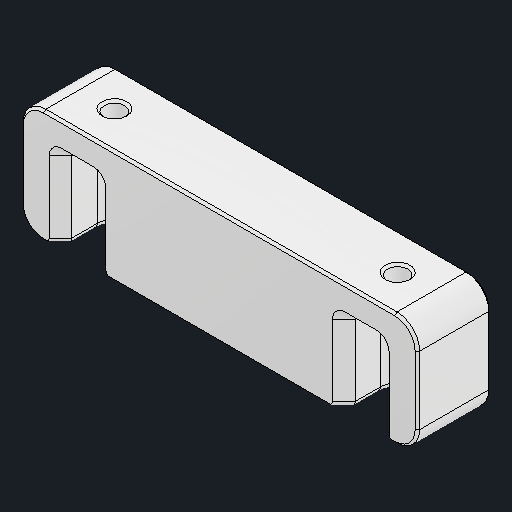
# Autodesk Inventor part: panel-mout
Saved by Autodesk Inventor 2026 (Build 300175050, 175E)
## iProperties
Created: 2026-03-04
Part Number: panel-mout
Material: ABS Plastic
Document SubType Name: Modeling
Designer: kuzmin
Density: 1.06 g/cm^3
Appearance: Smooth - White
Author: kuzmin
Autodesk Inventor part; units mm, degrees
ref_plane "YZ Plane" through (0, 0, 0) normal (1, 0, 0) x (0, 1, 0)
ref_plane "XZ Plane" through (0, 0, 0) normal (0, 1, 0) x (-1, 0, 0)
ref_plane "XY Plane" through (0, 0, 0) normal (0, 0, 1) x (1, 0, 0)
sketch "Sketch1" plane through (0, 0, 0) normal (0, 0, 1) x (1, 0, 0)
  line L0 (-35, 10) -> (35, 10)
  line L1 (35, 10) -> (35, -10)
  line L2 (35, -10) -> (-35, -10)
  line L3 (-35, -10) -> (-35, 10)
  point P0 (0, 0)
  point P1 (0, 10)
  point P2 (35, 0)
  dimension "d0" = 70
  dimension "d1" = 20
  constraints: 8 end point, 2 midpoint, 2 parallel, 1 horizontal, 1 horizontal alignment, 1 perpendicular, 1 vertical alignment
  measures "d0" distance of L0.start L0.end
  measures "d1" distance of L0.end L1.end
extrude "Extrusion1" add sketch "Sketch1" along normal mid plane 13
sketch "Sketch2" plane through (-35, 10, -6.5) normal (0, 1, 0) x (1, 0, 0)
  line L0 (10, -6.5) -> (60, -6.5) construction
  line L1 (0, 0) -> (70, 0) projected
  point P0 (35, -6.5)
  point P1 (35, 0)
  dimension "d4" = 50
  constraints: 2 coincident, 2 end point, 1 horizontal, 1 midpoint, 2 other
  measures "d4" distance of L0.start L0.end
hole "Hole1" at (-25, 10, 0) at (25, 10, 0) direction (0, -1, 0) diameter 3.6 end through all counterbore diameter 6 counterbore depth 13.8
sketch "Sketch3" plane through (-35, 10, 6.5) normal (0, 1, 0) x (1, 0, 0)
  circle A0 centre (10, 6.5) radius 3 projected
  circle A1 centre (60, 6.5) radius 3 projected
  line L0 (7, 6.5) -> (7, 13)
  line L1 (0, 13) -> (70, 13) projected
  line L2 (13, 6.5) -> (13, 13)
  line L3 (57, 6.5) -> (57, 13)
  line L4 (63, 6.5) -> (63, 13)
  point P0 (35, 6.5)
  constraints: 8 end point, 4 point on circle, 4 point on line, 3 parallel, 1 vertical
extrude "Extrusion2" cut sketch "Sketch3" against normal up to surface (13.8 mm away) contours A0 L0 L1 L2 | A1 L3 L1 L4
fillet "Fillet1" radius 0.2 6 edges at (-25, -3.8, 3) (-22, -3.8, -3.25) (-28, -3.8, -3.25) (25, -3.8, 3) (28, -3.8, -3.25) (22, -3.8, -3.25)
chamfer "Chamfer1" distance 2 angle 45 10 edges at (-28, 3.2, -6.5) (-27.9414, -3.7414, -6.5) (-25, -3.8, -6.5) (-22.0586, -3.7414, -6.5) (-22, 3.2, -6.5) (25, -3.8, -6.5) (27.9414, -3.7414, -6.5) (28, 3.2, -6.5) (22.0586, -3.7414, -6.5) (22, 3.2, -6.5)
fillet "Fillet2" radius 4 4 edges at (-35, 10, 0) (35, 10, 0) (35, -10, 0) (-35, -10, 0)
chamfer "Chamfer2" distance 0.4 angle 45 4 edges at (-25, -10, -1.8) (25, -10, -1.8) (25, -3.8, -1.8) (-25, -3.8, -1.8)
chamfer "Chamfer3" distance 0.4 angle 45 18 edges at (0, -10, -6.5) (-33.8284, -8.8284, -6.5) (-35, 0, -6.5) (-33.8284, 8.8284, -6.5) (-30.5, 10, -6.5) (33.8284, -8.8284, -6.5) (35, 0, -6.5) (33.8284, 8.8284, -6.5) (30.5, 10, -6.5) (0, 10, -6.5) (0, 10, 6.5) (-33.8284, 8.8284, 6.5) (-35, 0, 6.5) (-33.8284, -8.8284, 6.5) (0, -10, 6.5) (33.8284, -8.8284, 6.5) (35, 0, 6.5) (33.8284, 8.8284, 6.5)
fillet "Fillet3" radius 1 10 edges at (25, 10, 3) (28, 10, -2.25) (22, 10, -2.25) (-25, 10, 3) (-28, 10, -2.25) (-22, 10, -2.25) (-28.8, 10, -5.3) (-21.2, 10, -5.3) (21.2, 10, -5.3) (28.8, 10, -5.3)
move or copy body "Move Body1" bodies to move or copy 1 copy no rotation origin (0, 0, 0) rotation axis (1, 0, 0) rotation angle 180
body "Solid1"
